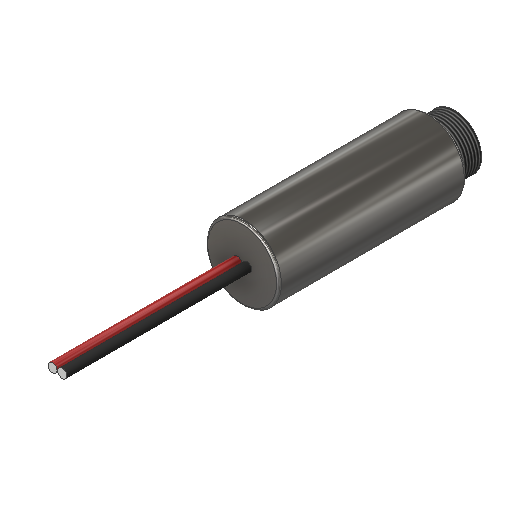
# Autodesk Inventor part: COTS_GENERIC_Engraving_laser
Saved by Autodesk Inventor 2026.1 (Build 301233000, 233)
## iProperties
Created: 2018-08-01
Part Number: COTS_GENERIC_Engraving_laser
Material: Generic
Document SubType Name: Modeling
Designer: Andrzej
Density: 1 g/cm^3
Appearance: Default
Author: Andrzej
Autodesk Inventor part; units mm, degrees
ref_plane "YZ Plane" through (0, 0, 0) normal (1, 0, 0) x (0, 1, 0)
ref_plane "XZ Plane" through (0, 0, 0) normal (0, 1, 0) x (-1, 0, 0)
ref_plane "XY Plane" through (0, 0, 0) normal (0, 0, 1) x (1, 0, 0)
sketch "Sketch1" plane through (0, 0, 0) normal (0, 0, 1) x (1, 0, 0)
  circle A0 centre (0, 0) radius 6
  dimension "d0" = 12
  constraints: 1 centre point, 1 coincident
  measures "d0" diameter of A0
extrude "Extrusion1" add sketch "Sketch1" along normal blind 30.5
sketch "Sketch2" plane through (0, 0, 30.5) normal (0, 0, 1) x (1, 0, 0)
  circle A0 centre (-0.8, 0) radius 0.75
  circle A1 centre (0.8, 0) radius 0.75
  circle A2 centre (0, 0) radius 1.75
  dimension "d3" = 1.5
  dimension "d4" = 1.5
  dimension "d5" = 1.6
  dimension "d6" = 0.8
  dimension "d7" = 3.5
  constraints: 3 centre point, 1 coincident
  measures "d3" diameter of A0
  measures "d4" diameter of A1
  measures "d5" distance of A1.centre A0.centre
  measures "d6" distance of point (0, 0) A1.centre
  measures "d7" diameter of A2
extrude "Extrusion2" add sketch "Sketch2" along normal blind 30 contours A0 | A1
sketch "Sketch3" plane through (0, 0, 0) normal (0, 0, -1) x (-1, 0, 0)
  circle A0 centre (0, 0) radius 4.4
  dimension "d10" = 8.8
  constraints: 1 centre point, 1 coincident
  measures "d10" diameter of A0
extrude "Extrusion3" add sketch "Sketch3" along normal blind 4
sketch "Sketch4" plane through (0, 0, -4) normal (0, 0, -1) x (-1, 0, 0)
  circle A0 centre (0, 0) radius 2.5
  dimension "d13" = 5
  constraints: 1 centre point, 1 coincident
  measures "d13" diameter of A0
extrude "Extrusion4" cut sketch "Sketch4" against normal blind 2
chamfer "Chamfer1" distance 1 angle 45 1 edges at (2.5, 0, -4)
thread "Thread1" size "M9x0.5" class "6g" standard "ANSI Metric M Profile" full length
fillet "Fillet1" radius 0.4 2 edges at (-6, 0, 30.5) (-6, 0, 0)
equation "\"d6\" = 0.5 * d5"
body "Solid1"
